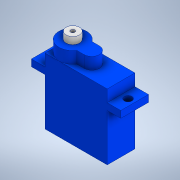
# Autodesk Inventor part: 9g-servo
Saved by Autodesk Inventor 2020 (Build 240168000, 168)
## iProperties
Created: 2020-11-06
Part Number: 9g-servo
Material: Generic
Document SubType Name: Modeling
Designer: alnwlsn
Density: 1 g/cm^3
Appearance: Default
Author: alnwlsn
Autodesk Inventor part; units mm, degrees
ref_plane "YZ Plane" through (0, 0, 0) normal (1, 0, 0) x (0, 1, 0)
ref_plane "XZ Plane" through (0, 0, 0) normal (0, 1, 0) x (-1, 0, 0)
ref_plane "XY Plane" through (0, 0, 0) normal (0, 0, 1) x (1, 0, 0)
sketch "Sketch1" plane through (0, 0, 0) normal (0, 0, 1) x (1, 0, 0)
  line L0 (0, 0) -> (22.45, 0)
  line L1 (22.45, 0) -> (22.45, 23.75)
  line L2 (22.45, 23.75) -> (0, 23.75)
  line L3 (0, 23.75) -> (0, 0)
  line L4 (-4.9, 19.45) -> (27.35, 19.45)
  line L5 (27.35, 19.45) -> (27.35, 17)
  line L6 (27.35, 17) -> (-4.9, 17)
  line L7 (-4.9, 17) -> (-4.9, 19.45)
  point P0 (0, 19.45)
  point P1 (0, 17)
  point P2 (22.45, 17)
  point P3 (22.45, 19.45)
  dimension "d0" = 23.75
  dimension "d1" = 22.45
  dimension "d2" = 2.45
  dimension "d3" = 17
  dimension "d4" = 4.9
  dimension "d5" = 4.9
  constraints: 16 end point, 4 parallel, 2 horizontal, 2 perpendicular
  measures "d0" distance between parallel lines of L0 L2
  measures "d1" distance between parallel lines of L1 L3
  measures "d2" distance between parallel lines of L6 L4
  measures "d3" distance between parallel lines of L0 L6
  measures "d4" distance between parallel lines of L1 L5
  measures "d5" distance between parallel lines of L3 L7
extrude "Extrusion1" add sketch "Sketch1" along normal blind 10
sketch "Sketch2" plane through (22.45, 19.45, 0) normal (0, 1, 0) x (1, 0, 0)
  line L0 (-27.35, 0) -> (-27.35, -10) projected
  line L1 (-27.35, -5) -> (4.9, -5) construction
  line L2 (4.9, 0) -> (4.9, -10) projected
  circle A0 centre (-24.975, -5) radius 1.385
  circle A1 centre (2.525, -5) radius 1.385
  circle A2 centre (-24.975, -5) radius 2.375 construction
  circle A3 centre (2.525, -5) radius 2.375 construction
  line L3 (4.9, 0) -> (4.9, -10) projected
  point P0 (-22.45, 0)
  dimension "d8" = 2.77
  dimension "d9" = 27.5
  constraints: 4 centre point, 2 coincident, 2 end point, 2 equal radius, 2 midpoint, 2 point on line, 2 tangent, 1 horizontal
  measures "d8" diameter of A0
  measures "d9" distance of A1.centre A0.centre
extrude "Extrusion2" cut sketch "Sketch2" against normal blind 10
sketch "Sketch3" plane through (0, 23.75, 0) normal (0, 1, 0) x (1, 0, 0)
  arc A0 (9.1758, -2.25) -> (9.1758, -7.75) centre (5, -5) ccw
  line L0 (22.45, 0) -> (0, 0) projected
  line L1 (0, 0) -> (0, -10) projected
  line L2 (22.45, -10) -> (0, -10) projected
  arc A1 (11.85, -7.75) -> (11.85, -2.25) centre (11.85, -5) ccw
  line L3 (14.6, -9.3785) -> (14.6, -0.6215) construction
  line L4 (11.85, -5) -> (0, -5) construction
  line L5 (0, 0) -> (0, -10) projected
  line L6 (11.85, -7.75) -> (9.1758, -7.75)
  line L7 (11.85, -2.25) -> (9.1758, -2.25)
  dimension "d12" = 5.5
  dimension "d13" = 14.6
  constraints: 8 end point, 6 tangent, 5 point on circle, 3 horizontal, 2 centre point, 1 midpoint, 1 vertical
  measures "d12" diameter of A1
  measures "d13" distance between parallel lines of L1 L3
extrude "Extrusion3" add sketch "Sketch3" along normal blind 4.3 contours L7 A1 L6 A0
sketch "Sketch4" plane through (0, 28.05, 0) normal (0, 1, 0) x (1, 0, 0)
  arc A0 (5, 0) -> (0, -5) centre (5, -5) ccw projected
  circle A1 centre (5, -5) radius 2.42
  circle A2 centre (5, -5) radius 0.75
  point P0 (0, 0)
  dimension "d16" = 4.84
  dimension "d17" = 1.5
  constraints: 2 centre point, 2 coincident
  measures "d16" diameter of A1
  measures "d17" diameter of A2
extrude "Extrusion4" add sketch "Sketch4" along normal blind 2.55
body "Solid1"
